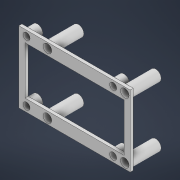
# Autodesk Inventor part: Adapter_Spannungswandler_v2
Saved by Autodesk Inventor 2021 (Build 250183000, 183)
## iProperties
Created: 2021-02-07
Part Number: Adapter_Spannungswandler_v2
Material: Generisch
Document SubType Name: Modeling
Designer: Ctroi
Density: 1 g/cm^3
Appearance: Vorgabe
Author: Ctroi
## iProperties of the stored document _3D-Druck.ipt
Created: 2021-02-08
Part Number: _3D-Druck
Material: Generisch
Document SubType Name: Modeling
Designer: Ctroi
Density: 1 g/cm^3
Appearance: Vorgabe
Author: Ctroi
Autodesk Inventor part; units mm, degrees
ref_plane "YZ Plane" through (0, 0, 0) normal (1, 0, 0) x (0, 1, 0)
ref_plane "XZ Plane" through (0, 0, 0) normal (0, 1, 0) x (-1, 0, 0)
ref_plane "XY Plane" through (0, 0, 0) normal (0, 0, 1) x (1, 0, 0)
sketch "Skizze1" plane through (0, 0, 0) normal (0, 0, 1) x (1, 0, 0)
  line L0 (-28.5, 23) -> (28.5, 23)
  line L1 (28.5, 23) -> (28.5, -23)
  line L2 (28.5, -23) -> (-28.5, -23)
  line L3 (-28.5, -23) -> (-28.5, 23)
  line L4 (0, 32.2) -> (0, -32.2) projected
  line L5 (-39.9, 0) -> (39.9, 0) projected
  point P0 (0, 0)
  point P1 (0, 23)
  point P2 (-28.5, 0)
  dimension "d0" = 57
  dimension "d1" = 46
  constraints: 8 end point, 2 parallel, 1 horizontal, 1 perpendicular, 2 other
  measures "d0" distance of L1.end L2.end
  measures "d1" distance of L0.end L1.end
extrude "Extrusion1" add sketch "Skizze1" along normal blind 2
sketch "Skizze2" plane through (0, 0, 0) normal (0, 0, -1) x (-1, 0, 0)
  circle A0 centre (25, -19.5) radius 3.5
  circle A1 centre (-25, -19.5) radius 3.5
  circle A2 centre (25, 19.5) radius 3.5
  circle A3 centre (-25, 19.5) radius 3.5
  line L0 (28.5, -23) -> (-28.5, -23) projected
  line L1 (28.5, 23) -> (28.5, -23) projected
  line L2 (-28.5, -23) -> (-28.5, 23) projected
  line L3 (-28.5, 23) -> (28.5, 23) projected
  point P0 (0, 0)
  dimension "d4" = 7
  dimension "d5" = 7
  dimension "d6" = 7
  dimension "d7" = 7
  dimension "d8" = 3.5
  dimension "d9" = 3.5
  dimension "d10" = 3.5
  dimension "d11" = 3.5
  dimension "d12" = 3.5
  dimension "d13" = 3.5
  dimension "d14" = 3.5
  dimension "d15" = 3.5
  constraints: 4 centre point
  measures "d4" diameter of A0
  measures "d5" diameter of A1
  measures "d6" diameter of A2
  measures "d7" diameter of A3
  measures "d8" distance from line of L0 A0.centre
  measures "d9" distance from line of L1 A0.centre
  measures "d10" distance from line of L0 A1.centre
  measures "d11" distance from line of L2 A1.centre
  measures "d12" distance from line of L1 A2.centre
  measures "d13" distance from line of L3 A2.centre
  measures "d14" distance from line of L3 A3.centre
  measures "d15" distance from line of L2 A3.centre
extrude "Extrusion2" add sketch "Skizze2" along normal blind 18 contours A0 | A2 | A1 | A3
sketch "Skizze3" plane through (0, 0, 2) normal (0, 0, 1) x (1, 0, 0)
  circle A0 centre (-25, 19.5) radius 2.75
  circle A1 centre (25, 19.5) radius 2.75
  circle A2 centre (-25, -19.5) radius 2.75
  circle A3 centre (25, -19.5) radius 2.75
  line L0 (28.5, 23) -> (-28.5, 23) projected
  line L1 (-28.5, 23) -> (-28.5, -23) projected
  line L2 (28.5, -23) -> (28.5, 23) projected
  line L3 (-28.5, -23) -> (28.5, -23) projected
  point P0 (0, 0)
  dimension "d18" = 5.5
  dimension "d19" = 5.5
  dimension "d20" = 5.5
  dimension "d21" = 5.5
  dimension "d22" = 3.5
  dimension "d23" = 3.5
  dimension "d24" = 3.5
  dimension "d25" = 3.5
  dimension "d26" = 3.5
  dimension "d27" = 3.5
  dimension "d28" = 3.5
  dimension "d29" = 3.5
  constraints: 4 centre point
  measures "d18" diameter of A0
  measures "d19" diameter of A1
  measures "d20" diameter of A2
  measures "d21" diameter of A3
  measures "d22" distance from line of L0 A0.centre
  measures "d23" distance from line of L1 A0.centre
  measures "d24" distance from line of L0 A1.centre
  measures "d25" distance from line of L2 A1.centre
  measures "d26" distance from line of L1 A2.centre
  measures "d27" distance from line of L3 A2.centre
  measures "d28" distance from line of L2 A3.centre
  measures "d29" distance from line of L3 A3.centre
extrude "Extrusion3" cut sketch "Skizze3" against normal blind 4 contours A0 | A1 | A2 | A3
sketch "Skizze4" plane through (-25, 19.5, -2) normal (0, 0, 1) x (1, 0, 0)
  circle A0 centre (0, 0) radius 2.75 projected
  circle A1 centre (0, 0) radius 1.6
  circle A2 centre (50, 0) radius 2.75 projected
  circle A3 centre (50, 0) radius 1.6
  circle A4 centre (50, -39) radius 2.75 projected
  circle A5 centre (50, -39) radius 1.6
  circle A6 centre (0, -39) radius 2.75 projected
  circle A7 centre (0, -39) radius 1.6
  point P0 (25, -19.5)
  dimension "d32" = 3.2
  dimension "d33" = 3.2
  dimension "d34" = 3.2
  dimension "d35" = 3.2
  constraints: 4 centre point, 4 coincident
  measures "d32" diameter of A1
  measures "d33" diameter of A3
  measures "d34" diameter of A5
  measures "d35" diameter of A7
extrude "Extrusion4" cut sketch "Skizze4" against normal up to surface (16 mm away) contours A1 | A3 | A5 | A7
sketch "Skizze5" plane through (-28.5, -23, 2) normal (-1, 0, 0) x (0, 0, 1)
  line L0 (-2, 0) -> (0, 0) projected
  line L1 (0, 0) -> (-2, 0)
  line L2 (-2, 0) -> (-2, 46)
  line L3 (-2, 46) -> (0, 46)
  line L4 (0, 46) -> (0, 0)
  point P0 (-2, 23)
  constraints: 8 end point, 2 parallel, 1 horizontal, 1 perpendicular
extrude "Extrusion5" add sketch "Skizze5" along normal blind 15
sketch "Skizze7" plane through (0, 0, 0) normal (0, 0, -1) x (-1, 0, 0)
  circle A0 centre (38.5, -19.5) radius 3.5
  line L0 (25, -23) -> (43.5, -23) projected
  line L1 (43.5, 23) -> (43.5, -23) projected
  circle A1 centre (38.5, 19.5) radius 3.5
  line L2 (25, 23) -> (43.5, 23) projected
  circle A2 centre (-17.5, 19.5) radius 3.5
  line L3 (-25, 23) -> (25, 23) projected
  line L4 (-28.5, -19.5) -> (-28.5, 19.5) projected
  circle A3 centre (-17.5, -19.5) radius 3.5
  line L5 (25, -23) -> (-25, -23) projected
  line L6 (-28.5, -23) -> (-28.5, -19.5) projected
  point P0 (0, 0)
  dimension "d53" = 7
  dimension "d54" = 3.5
  dimension "d55" = 5
  dimension "d56" = 7
  dimension "d57" = 5
  dimension "d58" = 3.5
  dimension "d59" = 7
  dimension "d60" = 3.5
  dimension "d61" = 11
  dimension "d62" = 7
  dimension "d63" = 3.5
  dimension "d64" = 11
  constraints: 4 centre point
  measures "d53" diameter of A0
  measures "d54" distance from line of L0 A0.centre
  measures "d55" distance from line of L1 A0.centre
  measures "d56" diameter of A1
  measures "d57" distance from line of L1 A1.centre
  measures "d58" distance from line of L2 A1.centre
  measures "d59" diameter of A2
  measures "d60" distance from line of L3 A2.centre
  measures "d61" distance from line of L4 A2.centre
  measures "d62" diameter of A3
  measures "d63" distance from line of L5 A3.centre
  measures "d64" distance from line of L6 A3.centre
extrude "Extrusion6" add sketch "Skizze7" along normal blind 5
sketch "Skizze6" plane through (0, 0, 2) normal (0, 0, 1) x (1, 0, 0)
  circle A0 centre (17.5, -19.5) radius 2.25
  circle A1 centre (17.5, 19.5) radius 2.25
  circle A2 centre (-38.5, -19.5) radius 2.25
  circle A3 centre (-38.5, 19.5) radius 2.25
  line L0 (-57.9, 0) -> (42.9, 0) projected
  line L1 (-43.5, -23) -> (-43.5, 23) projected
  point P0 (0, 0)
  dimension "d40" = 4.5
  dimension "d41" = 4.5
  dimension "d42" = 4.5
  dimension "d43" = 4.5
  dimension "d44" = 39
  dimension "d45" = 39
  dimension "d46" = 19.5
  dimension "d47" = 19.5
  dimension "d48" = 19.5
  dimension "d49" = 19.5
  dimension "d50" = 56
  dimension "d51" = 5
  constraints: 4 centre point
  measures "d40" diameter of A0
  measures "d41" diameter of A1
  measures "d42" diameter of A2
  measures "d43" diameter of A3
  measures "d44" distance of A1.centre A0.centre
  measures "d45" distance of A3.centre A2.centre
  measures "d46" distance from line of L0 A2.centre
  measures "d47" distance from line of L0 A3.centre
  measures "d48" distance from line of L0 A0.centre
  measures "d49" distance from line of L0 A1.centre
  measures "d50" distance of A0.centre A2.centre
  measures "d51" distance from line of L1 A2.centre
extrude "Extrusion7" cut sketch "Skizze6" against normal blind 6
sketch "Skizze8" plane through (0, 0, 2) normal (0, 0, 1) x (1, 0, 0)
  line L0 (-39.5, 15.5) -> (24.5, 15.5)
  line L1 (24.5, 15.5) -> (24.5, -15.5)
  line L2 (24.5, -15.5) -> (-39.5, -15.5)
  line L3 (-39.5, -15.5) -> (-39.5, 15.5)
  line L4 (28.5, -23) -> (28.5, 23) projected
  line L5 (28.5, 23) -> (-43.5, 23) projected
  line L6 (-43.5, -23) -> (-43.5, 23) projected
  line L7 (28.5, -23) -> (-43.5, -23) projected
  point P0 (0, 0)
  dimension "d69" = 4
  dimension "d70" = 7.5
  dimension "d71" = 4
  dimension "d72" = 7.5
  constraints: 8 end point, 2 parallel, 1 horizontal, 1 perpendicular
  measures "d69" distance between parallel lines of L4 L1
  measures "d70" distance between parallel lines of L5 L0
  measures "d71" distance between parallel lines of L6 L3
  measures "d72" distance between parallel lines of L7 L2
extrude "Extrusion8" cut sketch "Skizze8" against normal up to surface (2 mm away) contours L0 L1 L2 L3
